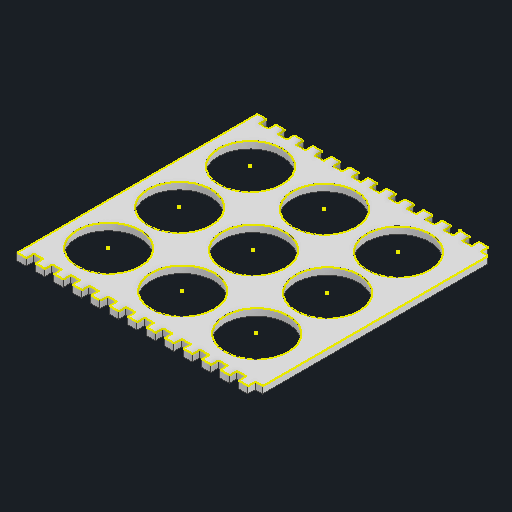
# Autodesk Inventor part: Top cover with groves
Saved by Autodesk Inventor 2023 (Build 270158030, 158C)
## iProperties
Created: 2022-06-21
Part Number: Top cover with groves
Material: Generic
Document SubType Name: Modeling
Designer: Simon
Density: 1 g/cm^3
Appearance: Default
Author: Simon
Autodesk Inventor part; units mm, degrees
ref_plane "YZ Plane" through (0, 0, 0) normal (1, 0, 0) x (0, 1, 0)
ref_plane "XZ Plane" through (0, 0, 0) normal (0, 1, 0) x (-1, 0, 0)
ref_plane "XY Plane" through (0, 0, 0) normal (0, 0, 1) x (1, 0, 0)
sketch "Sketch1" plane through (0, 0, 0) normal (0, 1, 0) x (-1, 0, 0)
  line L0 (-19, 126) -> (-19, 4)
  line L1 (-15, 126) -> (-19, 126)
  line L2 (-15, 126) -> (-15, 130)
  line L3 (-10, 130) -> (-15, 130)
  line L4 (-10, 126) -> (-10, 130)
  line L5 (-5, 126) -> (-10, 126)
  line L6 (-5, 126) -> (-5, 130)
  line L7 (0, 130) -> (-5, 130)
  line L8 (0, 126) -> (0, 130)
  line L9 (5, 126) -> (0, 126)
  line L10 (5, 126) -> (5, 130)
  line L11 (10, 130) -> (5, 130)
  line L12 (10, 126) -> (10, 130)
  line L13 (15, 126) -> (10, 126)
  line L14 (15, 126) -> (15, 130)
  line L15 (20, 130) -> (15, 130)
  line L16 (20, 126) -> (20, 130)
  line L17 (25, 126) -> (20, 126)
  line L18 (25, 126) -> (25, 130)
  line L19 (30, 130) -> (25, 130)
  line L20 (30, 126) -> (30, 130)
  line L21 (35, 126) -> (30, 126)
  line L22 (35, 126) -> (35, 130)
  line L23 (40, 130) -> (35, 130)
  line L24 (40, 126) -> (40, 130)
  line L25 (45, 126) -> (40, 126)
  line L26 (45, 126) -> (45, 130)
  line L27 (50, 130) -> (45, 130)
  line L28 (50, 126) -> (50, 130)
  line L29 (55, 126) -> (50, 126)
  line L30 (55, 126) -> (55, 130)
  line L31 (60, 130) -> (55, 130)
  line L32 (60, 126) -> (60, 130)
  line L33 (65, 126) -> (60, 126)
  line L34 (65, 126) -> (65, 130)
  line L35 (70, 130) -> (65, 130)
  line L36 (70, 126) -> (70, 130)
  line L37 (75, 126) -> (70, 126)
  line L38 (75, 126) -> (75, 130)
  line L39 (80, 130) -> (75, 130)
  line L40 (80, 126) -> (80, 130)
  line L41 (85, 126) -> (80, 126)
  line L42 (85, 126) -> (85, 130)
  line L43 (90, 130) -> (85, 130)
  line L44 (90, 126) -> (90, 130)
  line L45 (95, 126) -> (90, 126)
  line L46 (95, 126) -> (95, 130)
  line L47 (100, 130) -> (95, 130)
  line L48 (100, 126) -> (100, 130)
  line L49 (105, 126) -> (100, 126)
  line L50 (105, 126) -> (105, 130)
  line L51 (110, 130) -> (105, 130)
  line L52 (110, 126) -> (110, 130)
  line L53 (110, 65) -> (110, 126)
  line L54 (110, 65) -> (-15, 65)
  line L55 (110, 65) -> (235, 65) construction
  line L56 (-15, 65) -> (-19, 65)
  point P0 (0, 0)
  dimension "d0" = 180
  constraints: 114 end point, 1 collinear, 1 horizontal, 1 midpoint, 1 vertical
  measures "d0" angle of L54 L55
extrude "Extrusion1" add sketch "Sketch1" along normal blind 4
mirror "Mirror1" about plane through (19, 0, 65) normal (0, 0, -1) of "Extrusion1"
sketch "Sketch2" plane through (0, 4, 0) normal (0, 1, 0) x (1, 0, 0)
  circle A0 centre (-87.2711, -26.4814) radius 17.0835
  circle A1 centre (-7.1111, -26.4836) radius 17.0835
  circle A2 centre (-7.1122, -64.8602) radius 17.0835
  circle A3 centre (-7.1132, -103.2368) radius 17.0835
  circle A4 centre (-87.2732, -103.2346) radius 17.0835
  circle A5 centre (-87.2722, -64.858) radius 17.0835
  circle A6 centre (-47.1922, -64.8591) radius 17.0835
  circle A7 centre (-47.1932, -103.2357) radius 17.0835
  circle A8 centre (-47.1911, -26.4825) radius 17.0835
  line L0 (18.7695, -7.9481) -> (18.7695, -2.8242)
  line L1 (18.7695, -2.8242) -> (11.7661, -2.824)
  line L2 (11.7661, -2.824) -> (11.7661, 1.0564)
  line L3 (11.7661, 1.0564) -> (6.7661, 1.0564)
  line L4 (6.7661, 1.0564) -> (6.7661, -2.8239)
  line L5 (6.7661, -2.8239) -> (1.7661, -2.8238)
  line L6 (1.7661, -2.8238) -> (1.7661, 1.0564)
  line L7 (1.7661, 1.0564) -> (-3.2339, 1.0564)
  line L8 (-3.2339, 1.0564) -> (-3.2339, -2.8236)
  line L9 (-3.2339, -2.8236) -> (-8.2339, -2.8235)
  line L10 (-8.2339, -2.8235) -> (-8.2339, 1.0564)
  line L11 (-8.2339, 1.0564) -> (-13.2339, 1.0564)
  line L12 (-13.2339, 1.0564) -> (-13.2339, -2.8234)
  line L13 (-13.2339, -2.8234) -> (-18.2339, -2.8232)
  line L14 (-18.2339, -2.8232) -> (-18.2339, 1.0564)
  line L15 (-18.2339, 1.0564) -> (-23.2339, 1.0564)
  line L16 (-23.2339, 1.0564) -> (-23.2339, -2.8231)
  line L17 (-23.2339, -2.8231) -> (-28.2339, -2.8229)
  line L18 (-28.2339, -2.8229) -> (-28.2339, 1.0564)
  line L19 (-28.2339, 1.0564) -> (-33.2339, 1.0564)
  line L20 (-33.2339, 1.0564) -> (-33.2339, -2.8228)
  line L21 (-33.2339, -2.8228) -> (-38.2339, -2.8227)
  line L22 (-38.2339, -2.8227) -> (-38.2339, 1.0564)
  line L23 (-38.2339, 1.0564) -> (-43.2339, 1.0564)
  line L24 (-43.2339, 1.0564) -> (-43.2339, -2.8225)
  line L25 (-43.2339, -2.8225) -> (-48.2339, -2.8224)
  line L26 (-48.2339, -2.8224) -> (-48.2339, 1.0564)
  line L27 (-48.2339, 1.0564) -> (-53.2339, 1.0564)
  line L28 (-53.2339, 1.0564) -> (-53.2339, -2.8223)
  line L29 (-53.2339, -2.8223) -> (-58.2339, -2.8221)
  line L30 (-58.2339, -2.8221) -> (-58.2339, 1.0564)
  line L31 (-58.2339, 1.0564) -> (-63.2339, 1.0564)
  line L32 (-63.2339, 1.0564) -> (-63.2339, -2.822)
  line L33 (-63.2339, -2.822) -> (-68.2339, -2.8219)
  line L34 (-68.2339, -2.8219) -> (-68.2339, 1.0564)
  line L35 (-68.2339, 1.0564) -> (-73.2339, 1.0564)
  line L36 (-73.2339, 1.0564) -> (-73.2339, -2.8217)
  line L37 (-73.2339, -2.8217) -> (-78.2339, -2.8216)
  line L38 (-78.2339, -2.8216) -> (-78.2339, 1.0564)
  line L39 (-78.2339, 1.0564) -> (-83.2339, 1.0564)
  line L40 (-83.2339, 1.0564) -> (-83.2339, -2.8214)
  line L41 (-83.2339, -2.8214) -> (-88.2339, -2.8213)
  line L42 (-88.2339, -2.8213) -> (-88.2339, 1.0564)
  line L43 (-88.2339, 1.0564) -> (-93.2339, 1.0564)
  line L44 (-93.2339, 1.0564) -> (-93.2339, -2.8212)
  line L45 (-93.2339, -2.8212) -> (-98.2339, -2.821)
  line L46 (-98.2339, -2.821) -> (-98.2339, 1.0564)
  line L47 (-98.2339, 1.0564) -> (-103.2339, 1.0564)
  line L48 (-103.2339, 1.0564) -> (-103.2339, -2.8209)
  line L49 (-103.2339, -2.8209) -> (-108.2339, -2.8208)
  line L50 (-108.2339, -2.8208) -> (-108.2339, 1.0564)
  line L51 (-108.2339, 1.0564) -> (-113.2339, 1.0564)
  line L52 (-111.2338, -127.0687) -> (-106.2338, -127.0688)
  line L53 (-106.2338, -127.0688) -> (-106.2338, -130.9481)
  line L54 (-106.2338, -130.9481) -> (-101.2338, -130.9481)
  line L55 (-101.2338, -130.9481) -> (-101.2338, -127.069)
  line L56 (-101.2338, -127.069) -> (-96.2338, -127.0691)
  line L57 (-96.2338, -127.0691) -> (-96.2338, -130.9481)
  line L58 (-96.2338, -130.9481) -> (-91.2338, -130.9481)
  line L59 (-91.2338, -130.9481) -> (-91.2338, -127.0692)
  line L60 (-91.2338, -127.0692) -> (-86.2338, -127.0694)
  line L61 (-86.2338, -127.0694) -> (-86.2338, -130.9481)
  line L62 (-86.2338, -130.9481) -> (-81.2338, -130.9481)
  line L63 (-81.2338, -130.9481) -> (-81.2338, -127.0695)
  line L64 (-81.2338, -127.0695) -> (-76.2338, -127.0696)
  line L65 (-76.2338, -127.0696) -> (-76.2338, -130.9481)
  line L66 (-76.2338, -130.9481) -> (-71.2338, -130.9481)
  line L67 (-71.2338, -130.9481) -> (-71.2338, -127.0698)
  line L68 (-71.2338, -127.0698) -> (-66.2338, -127.0699)
  line L69 (-66.2338, -127.0699) -> (-66.2338, -130.9481)
  line L70 (-66.2338, -130.9481) -> (-61.2338, -130.9481)
  line L71 (-61.2338, -130.9481) -> (-61.2338, -127.07)
  line L72 (-61.2338, -127.07) -> (-56.2338, -127.0702)
  line L73 (-56.2338, -127.0702) -> (-56.2338, -130.9481)
  line L74 (-56.2338, -130.9481) -> (-51.2338, -130.9481)
  line L75 (-51.2338, -130.9481) -> (-51.2338, -127.0703)
  line L76 (-51.2338, -127.0703) -> (-46.2338, -127.0705)
  line L77 (-46.2338, -127.0705) -> (-46.2338, -130.9481)
  line L78 (-46.2338, -130.9481) -> (-41.2338, -130.9481)
  line L79 (-41.2338, -130.9481) -> (-41.2338, -127.0706)
  line L80 (-41.2338, -127.0706) -> (-36.2338, -127.0707)
  line L81 (-36.2338, -127.0707) -> (-36.2338, -130.9481)
  line L82 (-36.2338, -130.9481) -> (-31.2338, -130.9481)
  line L83 (-31.2338, -130.9481) -> (-31.2338, -127.0709)
  line L84 (-31.2338, -127.0709) -> (-26.2338, -127.071)
  line L85 (-26.2338, -127.071) -> (-26.2338, -130.9481)
  line L86 (-26.2338, -130.9481) -> (-21.2338, -130.9481)
  line L87 (-21.2338, -130.9481) -> (-21.2338, -127.0711)
  line L88 (-21.2338, -127.0711) -> (-16.2338, -127.0713)
  line L89 (-16.2338, -127.0713) -> (-16.2338, -130.9481)
  line L90 (-16.2338, -130.9481) -> (-11.2338, -130.9481)
  line L91 (-11.2338, -130.9481) -> (-11.2338, -127.0714)
  line L92 (-11.2338, -127.0714) -> (-6.2338, -127.0715)
  line L93 (-6.2338, -127.0715) -> (-6.2338, -130.9481)
  line L94 (-6.2338, -130.9481) -> (-1.2338, -130.9481)
  line L95 (-1.2338, -130.9481) -> (-1.2338, -127.0717)
  line L96 (-1.2338, -127.0717) -> (3.7662, -127.0718)
  line L97 (3.7662, -127.0718) -> (3.7662, -130.9481)
  line L98 (3.7662, -130.9481) -> (8.7662, -130.9481)
  line L99 (8.7662, -130.9481) -> (8.7662, -127.072)
  line L100 (8.7662, -127.072) -> (13.7662, -127.0721)
  line L101 (13.7662, -127.0721) -> (13.7662, -130.9481)
  line L102 (13.7662, -130.9481) -> (18.7662, -130.9481)
  line L103 (18.7662, -130.9481) -> (18.7662, -122.9481)
  line L104 (18.7662, -122.9481) -> (14.9302, -122.9481)
  line L105 (14.9302, -122.9481) -> (14.9304, -117.9481)
  line L106 (14.9304, -117.9481) -> (18.7665, -117.9481)
  line L107 (18.7665, -117.9481) -> (18.7665, -112.9481)
  line L108 (18.7665, -112.9481) -> (14.9305, -112.9481)
  line L109 (14.9305, -112.9481) -> (14.9306, -107.9481)
  line L110 (14.9306, -107.9481) -> (18.7668, -107.9481)
  line L111 (18.7668, -107.9481) -> (18.7668, -102.9481)
  line L112 (18.7668, -102.9481) -> (14.9308, -102.9481)
  line L113 (14.9308, -102.9481) -> (14.9309, -97.9481)
  line L114 (14.9309, -97.9481) -> (18.767, -97.9481)
  line L115 (18.767, -97.9481) -> (18.767, -92.9481)
  line L116 (18.767, -92.9481) -> (14.931, -92.9481)
  line L117 (14.931, -92.9481) -> (14.9312, -87.9481)
  line L118 (14.9312, -87.9481) -> (18.7673, -87.9481)
  line L119 (18.7673, -87.9481) -> (18.7673, -82.9481)
  line L120 (18.7673, -82.9481) -> (14.9313, -82.9481)
  line L121 (14.9313, -82.9481) -> (14.9314, -77.9481)
  line L122 (14.9314, -77.9481) -> (18.7676, -77.9481)
  line L123 (18.7676, -77.9481) -> (18.7676, -72.9481)
  line L124 (18.7676, -72.9481) -> (14.9316, -72.9481)
  line L125 (14.9316, -72.9481) -> (14.9317, -67.9481)
  line L126 (14.9317, -67.9481) -> (18.7679, -67.9481)
  line L127 (18.7679, -67.9481) -> (18.7679, -62.9481)
  line L128 (18.7679, -62.9481) -> (14.9319, -62.9481)
  line L129 (14.9319, -62.9481) -> (14.932, -57.9481)
  line L130 (14.932, -57.9481) -> (18.7681, -57.9481)
  line L131 (18.7681, -57.9481) -> (18.7681, -52.9481)
  line L132 (18.7681, -52.9481) -> (14.9321, -52.9481)
  line L133 (14.9321, -52.9481) -> (14.9323, -47.9481)
  line L134 (14.9323, -47.9481) -> (18.7684, -47.9481)
  line L135 (18.7684, -47.9481) -> (18.7684, -42.9481)
  line L136 (18.7684, -42.9481) -> (14.9324, -42.9481)
  line L137 (14.9324, -42.9481) -> (14.9325, -37.9481)
  line L138 (14.9325, -37.9481) -> (18.7687, -37.9481)
  line L139 (18.7687, -37.9481) -> (18.7687, -32.9481)
  line L140 (18.7687, -32.9481) -> (14.9327, -32.9481)
  line L141 (14.9327, -32.9481) -> (14.9328, -27.9481)
  line L142 (14.9328, -27.9481) -> (18.7689, -27.9481)
  line L143 (18.7689, -27.9481) -> (18.7689, -22.9481)
  line L144 (18.7689, -22.9481) -> (14.9329, -22.9481)
  line L145 (14.9329, -22.9481) -> (14.9331, -17.9481)
  line L146 (14.9331, -17.9481) -> (18.7692, -17.9481)
  line L147 (18.7692, -17.9481) -> (18.7692, -12.9481)
  line L148 (18.7692, -12.9481) -> (14.9332, -12.9481)
  line L149 (14.9332, -12.9481) -> (14.9334, -7.9481)
  line L150 (14.9334, -7.9481) -> (18.7695, -7.9481)
  point P0 (0, 0)
  point P1 (-47.2322, -64.8593)
  dimension "d3" = 132.0045
  dimension "d5" = 0
  dimension "d6" = 3.8804
  dimension "d7" = 47.0034
  dimension "d11" = 8
  constraints: 302 end point, 9 centre point
  measures "d3" distance between parallel lines of L102 L3
  measures "d6" distance of L1.end L2.end
  measures "d7" distance between parallel lines of L0 L18
  measures "d11" distance of L102.end L103.end
extrude "Extrusion2" cut sketch "Sketch2" against normal blind 6.5
sketch "Sketch3" plane through (0, 4, 0) normal (0, 1, 0) x (1, 0, 0)
  circle A0 centre (-47.1932, -103.2357) radius 17.0835 projected
  circle A1 centre (-87.2711, -26.4814) radius 17.0835 projected
  circle A2 centre (-47.1911, -26.4825) radius 17.0835 projected
  circle A3 centre (-47.1922, -64.8591) radius 17.0835 projected
  circle A4 centre (-7.1122, -64.8602) radius 17.0835 projected
  circle A5 centre (-87.2722, -64.858) radius 17.0835 projected
  circle A6 centre (-7.1111, -26.4836) radius 17.0835 projected
  circle A7 centre (-87.2732, -103.2346) radius 17.0835 projected
  circle A8 centre (-7.1132, -103.2368) radius 17.0835 projected
  line L0 (19, -126) -> (19, -4) projected
  line L1 (15, -4) -> (19, -4) projected
  line L2 (15, 0) -> (15, -4) projected
  line L3 (10, 0) -> (15, 0) projected
  line L4 (10, -4) -> (10, 0) projected
  line L5 (5, -4) -> (10, -4) projected
  line L6 (5, 0) -> (5, -4) projected
  line L7 (0, 0) -> (5, 0) projected
  line L8 (0, -4) -> (0, 0) projected
  line L9 (-5, -4) -> (0, -4) projected
  line L10 (-5, 0) -> (-5, -4) projected
  line L11 (-10, 0) -> (-5, 0) projected
  line L12 (-10, -4) -> (-10, 0) projected
  line L13 (-15, -4) -> (-10, -4) projected
  line L14 (-15, 0) -> (-15, -4) projected
  line L15 (-20, 0) -> (-15, 0) projected
  line L16 (-20, -4) -> (-20, 0) projected
  line L17 (-25, -4) -> (-20, -4) projected
  line L18 (-25, 0) -> (-25, -4) projected
  line L19 (-30, 0) -> (-25, 0) projected
  line L20 (-30, -4) -> (-30, 0) projected
  line L21 (-35, -4) -> (-30, -4) projected
  line L22 (-35, 0) -> (-35, -4) projected
  line L23 (-40, 0) -> (-35, 0) projected
  line L24 (-40, -4) -> (-40, 0) projected
  line L25 (-45, -4) -> (-40, -4) projected
  line L26 (-45, 0) -> (-45, -4) projected
  line L27 (-50, 0) -> (-45, 0) projected
  line L28 (-50, -4) -> (-50, 0) projected
  line L29 (-55, -4) -> (-50, -4) projected
  line L30 (-55, 0) -> (-55, -4) projected
  line L31 (-60, 0) -> (-55, 0) projected
  line L32 (-60, -4) -> (-60, 0) projected
  line L33 (-65, -4) -> (-60, -4) projected
  line L34 (-65, 0) -> (-65, -4) projected
  line L35 (-70, 0) -> (-65, 0) projected
  line L36 (-70, -4) -> (-70, 0) projected
  line L37 (-75, -4) -> (-70, -4) projected
  line L38 (-75, 0) -> (-75, -4) projected
  line L39 (-80, 0) -> (-75, 0) projected
  line L40 (-80, -4) -> (-80, 0) projected
  line L41 (-85, -4) -> (-80, -4) projected
  line L42 (-85, 0) -> (-85, -4) projected
  line L43 (-90, 0) -> (-85, 0) projected
  line L44 (-90, -4) -> (-90, 0) projected
  line L45 (-95, -4) -> (-90, -4) projected
  line L46 (-95, 0) -> (-95, -4) projected
  line L47 (-100, 0) -> (-95, 0) projected
  line L48 (-100, -4) -> (-100, 0) projected
  line L49 (-105, -4) -> (-100, -4) projected
  line L50 (-105, 0) -> (-105, -4) projected
  line L51 (-110, 0) -> (-105, 0) projected
  line L52 (-110, -130) -> (-110, 0) projected
  line L53 (-110, -130) -> (-105, -130) projected
  line L54 (-105, -130) -> (-105, -126) projected
  line L55 (-105, -126) -> (-100, -126) projected
  line L56 (-100, -126) -> (-100, -130) projected
  line L57 (-100, -130) -> (-95, -130) projected
  line L58 (-95, -130) -> (-95, -126) projected
  line L59 (-95, -126) -> (-90, -126) projected
  line L60 (-90, -126) -> (-90, -130) projected
  line L61 (-90, -130) -> (-85, -130) projected
  line L62 (-85, -130) -> (-85, -126) projected
  line L63 (-85, -126) -> (-80, -126) projected
  line L64 (-80, -126) -> (-80, -130) projected
  line L65 (-80, -130) -> (-75, -130) projected
  line L66 (-75, -130) -> (-75, -126) projected
  line L67 (-75, -126) -> (-70, -126) projected
  line L68 (-70, -126) -> (-70, -130) projected
  line L69 (-70, -130) -> (-65, -130) projected
  line L70 (-65, -130) -> (-65, -126) projected
  line L71 (-65, -126) -> (-60, -126) projected
  line L72 (-60, -126) -> (-60, -130) projected
  line L73 (-60, -130) -> (-55, -130) projected
  line L74 (-55, -130) -> (-55, -126) projected
  line L75 (-55, -126) -> (-50, -126) projected
  line L76 (-50, -126) -> (-50, -130) projected
  line L77 (-50, -130) -> (-45, -130) projected
  line L78 (-45, -130) -> (-45, -126) projected
  line L79 (-45, -126) -> (-40, -126) projected
  line L80 (-40, -126) -> (-40, -130) projected
  line L81 (-40, -130) -> (-35, -130) projected
  line L82 (-35, -130) -> (-35, -126) projected
  line L83 (-35, -126) -> (-30, -126) projected
  line L84 (-30, -126) -> (-30, -130) projected
  line L85 (-30, -130) -> (-25, -130) projected
  line L86 (-25, -130) -> (-25, -126) projected
  line L87 (-25, -126) -> (-20, -126) projected
  line L88 (-20, -126) -> (-20, -130) projected
  line L89 (-20, -130) -> (-15, -130) projected
  line L90 (-15, -130) -> (-15, -126) projected
  line L91 (-15, -126) -> (-10, -126) projected
  line L92 (-10, -126) -> (-10, -130) projected
  line L93 (-10, -130) -> (-5, -130) projected
  line L94 (-5, -130) -> (-5, -126) projected
  line L95 (-5, -126) -> (0, -126) projected
  line L96 (0, -126) -> (0, -130) projected
  line L97 (0, -130) -> (5, -130) projected
  line L98 (5, -130) -> (5, -126) projected
  line L99 (5, -126) -> (10, -126) projected
  line L100 (10, -126) -> (10, -130) projected
  line L101 (10, -130) -> (15, -130) projected
  line L102 (15, -130) -> (15, -126) projected
  line L103 (15, -126) -> (19, -126) projected
  point P0 (0, 0)
body "Solid1"
